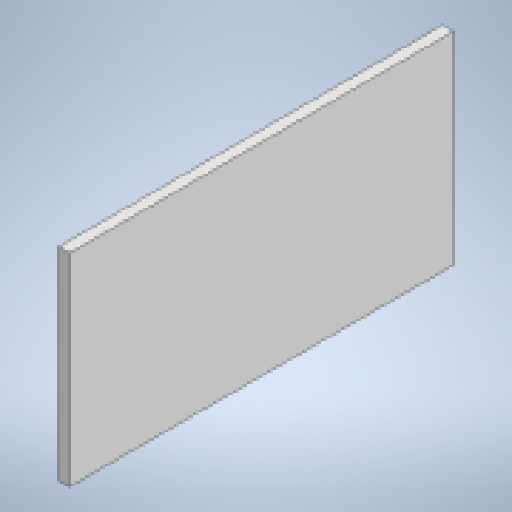
# Autodesk Inventor part: motorPlate
Saved by Autodesk Inventor 2023 (Build 270158000, 158)
## iProperties
Created: 2022-04-19
Part Number: motorPlate
Material: Generic
Document SubType Name: Modeling
Designer: carson
Density: 1 g/cm^3
Appearance: Default
Author: carson
Autodesk Inventor part; units mm, degrees
ref_plane "YZ Plane" through (0, 0, 0) normal (1, 0, 0) x (0, 1, 0)
ref_plane "XZ Plane" through (0, 0, 0) normal (0, 1, 0) x (-1, 0, 0)
ref_plane "XY Plane" through (0, 0, 0) normal (0, 0, 1) x (1, 0, 0)
sketch "Sketch1" plane through (0, 0, 0) normal (1, 0, 0) x (0, 1, 0)
  line L0 (-25, 50) -> (25, 50)
  line L1 (25, 50) -> (25, -50)
  line L2 (25, -50) -> (-25, -50)
  line L3 (-25, -50) -> (-25, 50)
  line L4 (-25, 50) -> (25, -50) construction
  line L5 (25, 50) -> (-25, -50) construction
  circle A0 centre (0, 40) radius 2.1
  circle A1 centre (0, 5) radius 2.1
  line L6 (0, 40) -> (0, 5)
  line L7 (25, 0) -> (-25, 0)
  circle A2 centre (0, -40) radius 2.1
  circle A3 centre (0, -5) radius 2.1
  point P0 (0, 0)
  point P1 (0, 50)
  dimension "d6" = 50
  dimension "d7" = 100
  dimension "d9" = 4.2
  dimension "d10" = 4.2
  dimension "d11" = 35
  dimension "d12" = 25
  dimension "d13" = 10
  constraints: 16 end point, 5 midpoint, 4 centre point, 3 parallel, 2 symmetric about line, 1 horizontal, 1 perpendicular, 2 other
  measures "d6" distance of L1.end L2.end
  measures "d7" distance of L0.end L1.end
  measures "d9" diameter of A0
  measures "d10" diameter of A1
  measures "d11" distance of L6.end L6.start
  measures "d12" distance from line of L1 L6.start
  measures "d13" distance of point (0, 50) L6.start
extrude "Extrusion2" add sketch "Sketch1" along normal blind 3
equation "\"d12\" = 0.5 * d6"
body "Solid2"
